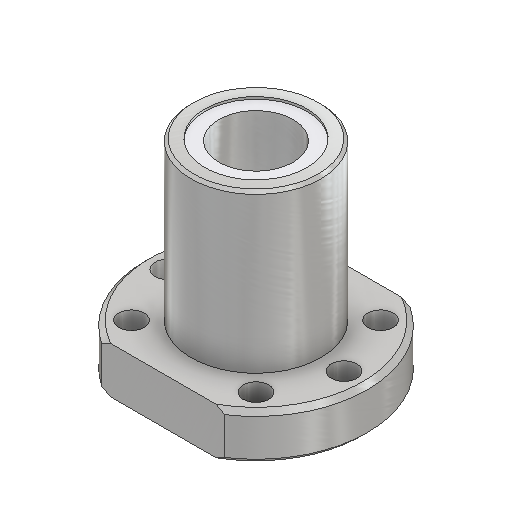
# Autodesk Inventor part: COTS_GENERIC_SFU1605_Ball_Screw_Nut
Saved by Autodesk Inventor 2026.1 (Build 301233000, 233)
## iProperties
Created: 2016-03-26
Part Number: COTS_GENERIC_SFU1605_Ball_Screw_Nut
Material: Ogólny
Document SubType Name: Modeling
Designer: Andrzej
Density: 1 g/cm^3
Appearance: Obrobione - aluminium
Mass: 27.0284 g
Surface Area: 102.295 cm^2
Volume: 27.0284 cm^3
Author: Andrzej
Autodesk Inventor part; units mm, degrees
ref_plane "YZ Plane" through (0, 0, 0) normal (1, 0, 0) x (0, 1, 0)
ref_plane "XZ Plane" through (0, 0, 0) normal (0, 1, 0) x (-1, 0, 0)
ref_plane "XY Plane" through (0, 0, 0) normal (0, 0, 1) x (1, 0, 0)
sketch "Szkic1" plane through (0, 0, 0) normal (0, 0, 1) x (1, 0, 0)
  circle A0 centre (0, 0) radius 14
  dimension "d0" = 28
  constraints: 1 centre point, 1 coincident
  measures "d0" diameter of A0
extrude "Wyciągnięcie proste1" add sketch "Szkic1" along normal blind 34
sketch "Szkic2" plane through (0, 0, 0) normal (0, 0, -1) x (-1, 0, 0)
  line L0 (13.2665, -20) -> (-13.2665, -20)
  line L1 (-13.2665, 20) -> (13.2665, 20)
  arc A0 (-13.2665, 20) -> (-13.2665, -20) centre (0, 0) ccw
  arc A1 (13.2665, -20) -> (13.2665, 20) centre (0, 0) ccw
  dimension "d18" = 20
  dimension "d19" = 20
  dimension "d20" = 24
  constraints: 4 end point, 4 point on circle, 2 centre point, 2 horizontal
  measures "d18" distance from line of L0 A0.centre
  measures "d19" distance from line of L1 A0.centre
  measures "d20" radius of A1
extrude "Wyciągnięcie proste2" add sketch "Szkic2" along normal blind 10
sketch "Szkic3" plane through (0, 0, 34) normal (0, 0, 1) x (1, 0, 0)
  circle A0 centre (0, 0) radius 8
  circle A1 centre (0, 0) radius 11
  dimension "d9" = 16
  dimension "d10" = 3
  constraints: 2 centre point, 1 coincident
  measures "d9" diameter of A0
  measures "d10" radial gap between concentric circles of A0 A1
extrude "Wyciągnięcie proste3" cut sketch "Szkic3" against normal up to surface (44 mm away) contours A0
extrude "Wyciągnięcie proste4" cut sketch "Szkic3" against normal blind 0.5
sketch "Szkic4" plane through (0, 0, -10) normal (0, 0, -1) x (-1, 0, 0)
  circle A0 centre (0, 0) radius 8 projected
  circle A1 centre (0, 0) radius 11
  circle A2 centre (0, 0) radius 19
  line L0 (-13.435, -13.435) -> (0, 0)
  line L1 (0, 0) -> (13.435, 13.435)
  line L2 (0, 0) -> (13.435, -13.435)
  line L3 (0, 0) -> (-13.435, 13.435)
  line L4 (-27.1999, 0) -> (26.3201, 0)
  arc A3 (-13.2665, 20) -> (-13.2665, -20) centre (0, 0) ccw projected
  line L5 (-13.2665, -20) -> (13.2665, -20) projected
  arc A4 (13.2665, -20) -> (13.2665, 20) centre (0, 0) ccw projected
  line L6 (13.2665, 20) -> (-13.2665, 20) projected
  point P0 (-19, 0)
  point P1 (19, 0)
  dimension "d15" = 3
  dimension "d23" = 19
  dimension "d28" = 38
  dimension "d29" = 45
  dimension "d30" = 45
  dimension "d31" = 45
  dimension "d32" = 45
  constraints: 10 end point, 5 point on circle, 2 centre point, 1 coincident, 1 horizontal, 1 point on line
  measures "d15" radial gap between concentric circles of A0 A1
  measures "d23" distance of point (-19, 0) point (0, 0)
  measures "d28" diameter of A2
  measures "d29" angle of L4 L3
  measures "d30" angle of L4 L0
  measures "d31" angle of L4 L2
  measures "d32" angle of L1 L4
extrude "Wyciągnięcie proste5" cut sketch "Szkic4" against normal blind 0.5 contours L4 A1 L2 A0 | A0 L1 A1 L4 | A0 L3 A1 L1 | L2 A1 L0 A0 | A0 L4 A1 L3 | L0 A1 L4 A0
hole "Otwór1" at (13.435, -13.435, -10) at (19, 0, -10) at (13.435, 13.435, -10) at (-13.435, 13.435, -10) at (-19, 0, -10) at (-13.435, -13.435, -10) direction (0, 0, 1) diameter 5.5 end through all
chamfer "Faza1" distance 1 angle 45 4 edges at (-24, 0, 0) (-24, 0, -10) (24, 0, 0) (24, 0, -10)
chamfer "Faza2" distance 0.6 angle 45 1 edges at (-14, 0, 34)
